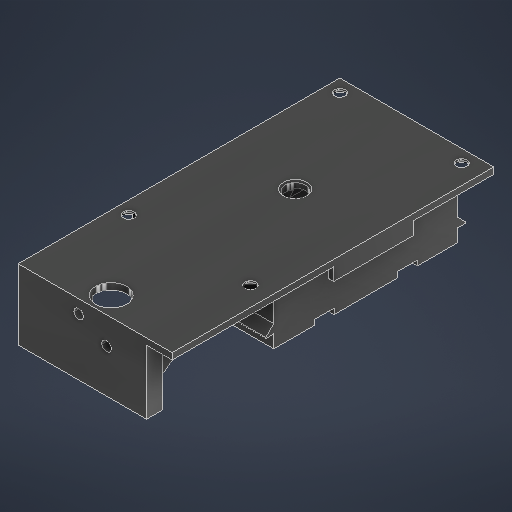
# Autodesk Inventor part: Flex holder Base V1
Saved by Autodesk Inventor 2027 (Build 310192060, 192F)
## iProperties
Created: 2025-07-06
Part Number: Flex holder Base V1
Material: Generic
Document SubType Name: Modeling
Designer: Caleb Fangmeier
Density: 1 g/cm^3
Appearance: Dark Gray
Author: Caleb Fangmeier
Autodesk Inventor part; units mm, degrees
ref_plane "XZ Plane" through (0, 0, 0) normal (0, 1, 0) x (-1, 0, 0)
ref_plane "XY Plane" through (0, 0, 0) normal (0, 0, 1) x (1, 0, 0)
sketch "Sketch1" plane through (0, 0, 0) normal (0, 1, 0) x (-1, 0, 0)
  line L0 (-22.05, -28.75) -> (22.05, -28.75)
  line L1 (22.05, -28.75) -> (22.05, 28.75)
  line L2 (22.05, 28.75) -> (-22.05, 28.75)
  line L3 (-22.05, 28.75) -> (-22.05, -28.75)
  line L4 (-22.05, -28.75) -> (22.05, 28.75) construction
  line L5 (22.05, -28.75) -> (-22.05, 28.75) construction
  point P0 (0, 0)
  dimension "d0" = 44.1
  dimension "d1" = 57.5
  constraints: 12 end point, 2 midpoint, 2 parallel, 1 horizontal, 1 perpendicular
  measures "d0" distance of L1.end L2.end
  measures "d1" distance of L0.end L1.end
extrude "Extrusion1" add sketch "Sketch1" along normal blind 14
chamfer "Chamfer1" distance 2 angle 45 1 edges at (-22.05, 7, -28.75)
sketch "Sketch3" plane through (0, 0, 0) normal (0, -1, 0) x (1, 0, 0)
  line L0 (-9.91, 21.965) -> (6.78, 21.965) construction
  line L1 (-9.91, 26.1) -> (6.78, 26.1)
  line L2 (6.78, 17.83) -> (-9.91, 17.83)
  arc A0 (-9.91, 26.1) -> (-9.91, 17.83) centre (-9.91, 21.965) ccw
  arc A1 (6.78, 17.83) -> (6.78, 26.1) centre (6.78, 21.965) ccw
  line L3 (-6.98, -22.52) -> (9.95, -22.52) construction
  line L4 (-6.98, -26.62) -> (9.95, -26.62)
  line L5 (9.95, -18.42) -> (-6.98, -18.42)
  arc A2 (-6.98, -18.42) -> (-6.98, -26.62) centre (-6.98, -22.52) ccw
  arc A3 (9.95, -26.62) -> (9.95, -18.42) centre (9.95, -22.52) ccw
  line L6 (22.05, -28.75) -> (-20.05, -28.75) projected
  line L7 (22.05, 28.75) -> (22.05, -28.75) projected
  line L8 (-22.05, -26.75) -> (-22.05, 28.75) projected
  line L9 (-22.05, 28.75) -> (22.05, 28.75) projected
  arc A4 (-4, 28.75) -> (4, 28.75) centre (0, 28.75) ccw
  arc A5 (4, -28.75) -> (-4, -28.75) centre (0, -28.75) ccw
  point P0 (0, 0)
  point P1 (-1.565, 21.965)
  point P2 (1.485, -22.52)
  point P3 (2.9962, 26.1)
  point P4 (-2.9962, 26.1)
  point P5 (-3.3857, -26.62)
  point P6 (3.3857, -26.62)
  dimension "d196" = 8.2
  dimension "d197" = 2.13
  dimension "d198" = 16.93
  dimension "d200" = 15.07
  dimension "d201" = 12.14
  dimension "d202" = 2.65
  dimension "d203" = 8.27
  dimension "d204" = 16.69
  dimension "d207" = 4
  dimension "d208" = 4
  constraints: 16 end point, 12 point on circle, 8 tangent, 6 centre point, 5 point on line, 3 midpoint, 3 parallel, 2 horizontal alignment, 1 horizontal
  measures "d196" distance between parallel lines of L5 L4
  measures "d197" distance between parallel lines of L4 L6
  measures "d198" distance of L3.start L3.end
  measures "d200" distance from line of L3.start L8
  measures "d201" distance from line of L8 L0.start
  measures "d202" distance between parallel lines of L9 L1
  measures "d203" distance between parallel lines of L2 L1
  measures "d204" distance of L0.start L0.end
  measures "d207" radius of A4
  measures "d208" radius of A5
extrude "Extrusion2" cut sketch "Sketch3" against normal through all contours L1 A4 A1 L2 A0 | A2 L5 A3 L4 A5
sketch "Sketch7" plane through (0, 14, 0) normal (0, 1, 0) x (1, 0, 0)
  line L0 (-22.05, 26.75) -> (-20.05, 28.75) projected
  line L1 (-22.05, 26.75) -> (-22.05, -28.75) projected
  line L2 (22.05, -28.75) -> (22.05, 28.75) projected
  line L3 (2.5, -21) -> (-2.5, -21)
  line L4 (-2.5, -21) -> (-2.5, 21)
  line L5 (-2.5, 21) -> (2.5, 21)
  line L6 (2.5, 21) -> (2.5, -21)
  line L7 (2.5, -21) -> (-2.5, 21) construction
  line L8 (-2.5, -21) -> (2.5, 21) construction
  line L9 (22.05, 28.75) -> (-20.05, 28.75) projected
  line L10 (-22.05, -28.75) -> (22.05, -28.75) projected
  point P0 (0, 0)
  dimension "d205" = 5
  dimension "d206" = 42
  dimension "d209" = 22.05
  dimension "d210" = 44.1
  dimension "d211" = 57.5
  dimension "d212" = 28.75
  constraints: 12 end point, 2 midpoint, 2 parallel, 1 horizontal, 1 perpendicular
  measures "d205" distance of L4.end L5.end
  measures "d206" distance of L3.end L4.end
  measures "d209" distance from line of L2 point (0, 0)
  measures "d210" distance of L1.end L2.start
  measures "d211" distance of L2.start L2.end
  measures "d212" distance from line of L10 point (0, 0)
extrude "Extrusion6" add sketch "Sketch7" along normal blind 2
sketch "Sketch8" plane through (0, 16, 0) normal (0, 1, 0) x (1, 0, 0)
  line L0 (-23.05, 36.6331) -> (-23.05, -63.5)
  line L1 (25.05, 37) -> (-23.05, 37)
  line L2 (-23.05, 37) -> (-23.05, -63.5)
  line L3 (-23.05, -63.5) -> (25.05, -63.5)
  line L4 (25.05, -63.5) -> (25.05, 37)
  line L5 (22.05, -28.75) -> (22.05, 28.75) projected
  line L6 (-22.05, 26.75) -> (-22.05, -28.75) projected
  line L7 (22.05, 28.75) -> (-20.05, 28.75) projected
  line L8 (-22.05, -28.75) -> (22.05, -28.75) projected
  point P0 (0, 0)
  point P1 (-23.05, 37)
  dimension "d79" = 3
  dimension "d80" = 1
  dimension "d81" = 8.25
  dimension "d82" = 34.75
  constraints: 10 end point, 2 parallel, 1 horizontal, 1 perpendicular
  measures "d79" distance between parallel lines of L4 L5
  measures "d80" distance between parallel lines of L0 L6
  measures "d81" distance between parallel lines of L1 L7
  measures "d82" distance between parallel lines of L3 L8
extrude "Extrusion7" add sketch "Sketch8" along normal blind 2
sketch "Sketch9" plane through (0, 16, 0) normal (0, -1, 0) x (1, 0, 0)
  point P0 (0, 0)
  point P1 (19, -33)
  point P2 (-19, -33)
  point P3 (19, 33)
  point P4 (-19, 33)
  dimension "d55" = 66
  dimension "d56" = 38
  dimension "d57" = 33
  dimension "d58" = 19
  constraints: 2 horizontal alignment, 2 vertical alignment
  measures "d55" distance of point (19, 33) point (19, -33)
  measures "d56" distance of point (-19, -33) point (19, -33)
  measures "d57" vertical distance of point (19, 33) point (0, 0)
  measures "d58" horizontal distance of point (19, -33) point (0, 0)
hole "Hole1" at (19, 16, -33) at (-19, 16, -33) at (19, 16, 33) at (-19, 16, 33) direction (0, 1, 0) diameter 3.4 end through all countersink diameter 6.3 countersink angle 90 clearance for "Flat Head Machine Screw" size "M3" standard "Ansi Metric M Profile"
sketch "Sketch10" plane through (0, 18, 0) normal (0, 1, 0) x (1, 0, 0)
  circle A0 centre (0, 0) radius 3.175
  circle A1 centre (-19, 33) radius 1.7 projected
  dimension "d74" = 6.35
  constraints: 1 centre point, 1 coincident
  measures "d74" diameter of A0
extrude "Extrusion8" cut sketch "Sketch10" against normal blind 4 contours A0
chamfer "Chamfer2" distance 1.5 distance2 0.6 3 edges at (3.0015, 14, 1.0352) (3.0015, 14, -1.0352) (-3.175, 14, 0) measured on face at (3.0015, 14.5, -1.0352) measured on face at (3.0015, 14.5, 1.0352) measured on face at (-3.175, 14.5, 0)
chamfer "Chamfer3" distance 0.5 angle 45 1 edges at (-3.175, 18, 0)
sketch "Sketch12" plane through (0, 16, 0) normal (0, -1, 0) x (1, 0, 0)
  line L0 (25.05, 63.5) -> (25.05, -37) projected
  line L1 (25.05, -12) -> (23.55, -12)
  line L2 (23.55, -12) -> (23.55, 13)
  line L3 (23.55, 13) -> (25.05, 13)
  line L4 (25.05, 13) -> (25.05, -12)
  line L5 (25.05, -37) -> (-23.05, -37) projected
  point P0 (0, 0)
  point P1 (23.05, -37)
  dimension "d92" = 1.5
  dimension "d93" = 25
  dimension "d94" = 25
  constraints: 8 end point, 2 parallel, 1 horizontal, 1 perpendicular, 1 point on line
  measures "d92" distance of L1.start L1.end
  measures "d93" distance between parallel lines of L1 L5
  measures "d94" distance between parallel lines of L1 L3
extrude "Extrusion10" add sketch "Sketch12" along normal blind 4
sketch "Sketch19" plane through (0, 0, 0) normal (0, -1, 0) x (1, 0, 0)
  line L0 (22.05, 28.75) -> (22.05, -28.75) projected
  line L1 (22.05, -16.1) -> (-12, -16.1)
  line L2 (-12, -16.1) -> (-12, -9.9)
  line L3 (-4.8, -9.9) -> (22.05, -9.9)
  line L4 (22.05, -9.9) -> (22.05, -16.1)
  line L5 (-12, -16.1) -> (-5.8, -16.1)
  line L6 (-5.8, -8.9) -> (-5.8, 8.9)
  line L7 (-5.8, 16.1) -> (-12, 16.1)
  line L8 (-12, 16.1) -> (-12, -16.1)
  line L9 (-12, 16.1) -> (22.05, 16.1)
  line L10 (22.05, 16.1) -> (22.05, 9.9)
  line L11 (22.05, 9.9) -> (-4.8, 9.9)
  line L12 (-12, 9.9) -> (-12, 16.1)
  arc A0 (-5.8, -8.9) -> (-4.8, -9.9) centre (-4.8, -8.9) ccw
  arc A1 (-4.8, 9.9) -> (-5.8, 8.9) centre (-4.8, 8.9) ccw
  point P0 (0, 0)
  point P1 (22.05, -9.9)
  dimension "d134" = 32.2
  dimension "d135" = 16.1
  dimension "d136" = 19.8
  dimension "d137" = 9.9
  dimension "d139" = 6.2
  dimension "d140" = 6.2
  dimension "d141" = 6.2
  dimension "d142" = 27.85
  dimension "d143" = 1
  dimension "d144" = 1
  constraints: 24 end point, 6 parallel, 6 point on line, 4 point on circle, 4 tangent, 3 horizontal, 3 perpendicular, 2 centre point
  measures "d134" distance of L7.end L1.end
  measures "d135" distance from line of L1 point (0, 0)
  measures "d136" distance between parallel lines of L3 L11
  measures "d137" distance from line of L3 point (0, 0)
  measures "d139" distance between parallel lines of L9 L11
  measures "d140" distance between parallel lines of L1 L3
  measures "d141" distance between parallel lines of L8 L6
  measures "d142" distance between parallel lines of L0 L6
  measures "d143" radius of A0
  measures "d144" radius of A1
extrude "Extrusion13" cut sketch "Sketch19" against normal blind 1.75 contours L0 L11 A1 L6 A0 L3 L1 L2 L8 L7 L9
sketch "Sketch20" plane through (0, 1.75, 0) normal (0, -1, 0) x (1, 0, 0)
  line L0 (-5.8, 8.9) -> (-5.8, -8.9) projected
  point P0 (0, 0)
  point P1 (-8.9, -13)
  point P2 (-8.9, 0)
  point P3 (-8.9, 13)
  point P4 (3.6, 13)
  point P5 (17.6, 13)
  point P6 (17.6, -13)
  point P7 (3.6, -13)
  dimension "d148" = 12.5
  dimension "d149" = 14
  dimension "d150" = 3.1
  dimension "d151" = 13
  dimension "d152" = 13
  constraints: 5 horizontal alignment, 4 vertical alignment
  measures "d148" distance of point (3.6, -13) point (-8.9, -13)
  measures "d149" distance of point (17.6, -13) point (3.6, -13)
  measures "d150" distance from line of point (-8.9, 0) L0
  measures "d151" distance of point (-8.9, -13) point (-8.9, 0)
  measures "d152" distance of point (-8.9, 13) point (-8.9, 0)
hole "Hole3" at (17.6, 1.75, 13) at (3.6, 1.75, 13) at (-8.9, 1.75, 13) at (-8.9, 1.75, 0) at (-8.9, 1.75, -13) at (3.6, 1.75, -13) at (17.6, 1.75, -13) direction (0, 1, 0) diameter 2.2 depth 5 counterbore diameter 3 counterbore depth 2
sketch "Sketch21" plane through (0, 0, 0) normal (0, -1, 0) x (1, 0, 0)
  line L0 (-12, 16.1) -> (22.05, 16.1) projected
  line L1 (22.05, 28.75) -> (22.05, 16.1) projected
  line L2 (-22.05, 28.75) -> (22.05, 28.75) projected
  line L3 (-22.05, -26.75) -> (-22.05, 28.75) projected
  line L4 (-20.05, -28.75) -> (-22.05, -26.75) projected
  line L5 (22.05, -28.75) -> (-20.05, -28.75) projected
  line L6 (22.05, -16.1) -> (22.05, -28.75) projected
  line L7 (22.05, -16.1) -> (-12, -16.1) projected
  line L8 (-12, -16.1) -> (-12, 16.1) projected
  point P0 (0, 0)
extrude "Extrusion14" cut sketch "Sketch21" against normal blind 0.15
ref_plane "Work Plane2" through (-20, 0, 0) normal (1, 0, 0) x (0, 1, 0)
sketch "Sketch13" plane through (0, 16, 0) normal (0, -1, 0) x (1, 0, 0)
  line L0 (-23.05, -37) -> (-23.05, 63.5) projected
  line L1 (-23.05, 63.5) -> (17.05, 63.5)
  line L2 (17.05, 63.5) -> (17.05, 58.5)
  line L3 (17.05, 58.5) -> (-23.05, 58.5)
  line L4 (-23.05, 58.5) -> (-23.05, 63.5)
  line L5 (25.05, 63.5) -> (25.05, 13) projected
  point P0 (0, 0)
  point P1 (-23.05, 37)
  dimension "d162" = 5
  dimension "d163" = 8
  constraints: 8 end point, 2 parallel, 1 horizontal, 1 perpendicular
  measures "d162" distance between parallel lines of L3 L1
  measures "d163" distance between parallel lines of L5 L2
extrude "Extrusion11" add sketch "Sketch13" along normal blind 20
sketch "Sketch16" plane through (-23.05, 18, 63.5) normal (0, 0, 1) x (1, 0, 0)
  line L0 (48.1, -2) -> (48.1, 0) projected
  line L1 (48.1, -22) -> (0, -22) projected
  line L2 (0, 0) -> (48.1, 0) projected
  point P0 (23.05, -18)
  point P1 (27.6, -8.5)
  point P2 (18.888, -4.13)
  dimension "d114" = 20.5
  dimension "d117" = 8.5
  dimension "d132" = 8.712
  dimension "d133" = 4.37
  measures "d114" distance from line of L0 point (27.6, -8.5)
  measures "d117" distance from line of L2 point (27.6, -8.5)
  measures "d132" horizontal distance of point (18.888, -4.13) point (27.6, -8.5)
  measures "d133" vertical distance of point (18.888, -4.13) point (27.6, -8.5)
hole "Hole2" at (4.55, 9.5, 63.5) at (-4.162, 13.87, 63.5) direction (0, 0, -1) diameter 2.2 depth 5 counterbore diameter 3 counterbore depth 2
sketch "Sketch23" plane through (-20, 0, 0) normal (1, 0, 0) x (0, 1, 0)
  line L0 (16, 58.5) -> (-4, 58.5) projected
  line L1 (2.1119, 58.5) -> (16, 39.8605)
  line L2 (16, -37) -> (16, 58.5) projected
  point P0 (0, 0)
  point P1 (16, 37)
  constraints: 2 end point, 2 point on line
extrude "Rib3" add sketch "Sketch23" along normal mid plane 2 rib yes fills toward (9.0961, 49.2101) open curves L1
pattern_linear "Rectangular Pattern2" count 2 spacing 34 along (1, 0, 0) of "Rib3"
sketch "Sketch25" plane through (22.05, 16, 28.75) normal (1, 0, 0) x (0, 0, -1)
  line L0 (57.5, -15.85) -> (57.5, 0) projected
  line L1 (57.5, -9.0216) -> (59.987, -11.5086)
  line L2 (57.5, -9.0216) -> (61.0172, -9.0216) construction
  line L3 (59.8456, -11.85) -> (57.5, -11.85)
  line L4 (44.85, -15.85) -> (57.5, -15.85) projected
  arc A0 (59.8456, -11.85) -> (59.987, -11.5086) centre (59.8456, -11.65) ccw
  line L5 (0, -15.85) -> (0, 0) projected
  line L6 (0, -9.0216) -> (-2.487, -11.5086)
  line L7 (0, -9.0216) -> (3.5172, -9.0216) construction
  line L8 (-2.3456, -11.85) -> (0, -11.85)
  arc A1 (-2.487, -11.5086) -> (-2.3456, -11.85) centre (-2.3456, -11.65) ccw
  line L9 (0, -15.85) -> (12.65, -15.85) projected
  point P0 (28.75, -16)
  point P1 (60.3284, -11.85)
  point P2 (-2.8284, -11.85)
  point P3 (57.5, -2)
  point P4 (0, -2)
  dimension "d186" = 4
  dimension "d187" = 45
  dimension "d188" = 4
  dimension "d189" = 0.2
  dimension "d190" = 4
  dimension "d191" = 135
  dimension "d192" = 0.2
  dimension "d193" = 4
  constraints: 12 end point, 8 point on line, 4 horizontal, 4 point on circle, 4 tangent, 2 centre point, 2 equal length
  measures "d186" distance of L1.start point (60.328, -11.85)
  measures "d187" angle of L1 L2
  measures "d188" distance between parallel lines of L3 L4
  measures "d189" radius of A0
  measures "d190" distance of L6.start point (-2.828, -11.85)
  measures "d191" angle of L6 L7
  measures "d192" radius of A1
  measures "d193" distance between parallel lines of L9 L8
extrude "Extrusion15" add sketch "Sketch25" against normal up to surface (42.1 mm away)
sketch "Sketch26" plane through (0, -4, 0) normal (0, -1, 0) x (1, 0, 0)
  circle A0 centre (0, 57.5) radius 4.8625
  line L0 (17.05, 63.5) -> (-23.05, 63.5) projected
  arc A1 (-2.9962, 26.1) -> (2.9962, 26.1) centre (0, 28.75) ccw projected
  point P0 (0, 0)
  dimension "d213" = 9.725
  dimension "d214" = 6
  constraints: 1 centre point, 1 vertical alignment
  measures "d213" diameter of A0
  measures "d214" distance from line of A0.centre L0
extrude "Extrusion16" cut sketch "Sketch26" against normal through all
equation "\"d208\" = d207"
equation "\"d209\" = 0.5 * d210"
equation "\"d212\" = 0.5 * d211"
equation "\"d57\" = 0.5 * d55"
equation "\"d58\" = 0.5 * d56"
equation "\"d135\" = 0.5 * d134"
equation "\"d137\" = 0.5 * d136"
equation "\"d141\" = d140"
equation "\"d152\" = d151"
body "Solid1"
